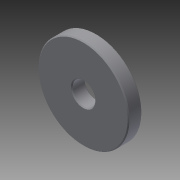
# Autodesk Inventor part: Magnet
Saved by Autodesk Inventor 2015 (Build 190159000, 159)
## iProperties
Created: 2015-01-06
Part Number: Magnet
Material: Generic
Document SubType Name: Modeling
Designer: ice
Density: 1 g/cm^3
Appearance: Default
Mass: 0.463342 g
Surface Area: 4.37557 cm^2
Volume: 0.463342 cm^3
Author: ice
Autodesk Inventor part; units mm, degrees
ref_plane "YZ Plane" through (0, 0, 0) normal (1, 0, 0) x (0, 1, 0)
ref_plane "XZ Plane" through (0, 0, 0) normal (0, 1, 0) x (-1, 0, 0)
ref_plane "XY Plane" through (0, 0, 0) normal (0, 0, 1) x (1, 0, 0)
sketch "Sketch1" plane through (0, 0, 0) normal (0, 1, 0) x (-1, 0, 0)
  circle A0 centre (0, 0) radius 2.5
  circle A1 centre (0, 0) radius 10
  dimension "d0" = 5
  dimension "d5" = 20
  constraints: 2 centre point, 1 coincident
  measures "d0" diameter of A0
  measures "d5" diameter of A1
extrude "Extrusion2" add sketch "Sketch1" along normal blind 3
chamfer "Chamfer1" distance 0.2 angle 45 4 edges at (10, 3, 0) (10, 0, 0) (2.5, 0, 0) (2.5, 3, 0)
body "Solid2"
